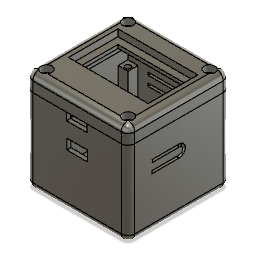
Digital Die v5 (Autodesk Fusion 360 design; units mm, degrees)
Autodesk Fusion 360 part; units mm, degrees
note: some values were not read from the file. Set by a fixed rule: which sketch regions a step uses.
sketch "Sketch1" plane through (0, 0, 0) normal (0, 1, 0) x (1, 0, 0)
  line L0 (0, 0) -> (38.1, 0)
  line L1 (38.1, 0) -> (38.1, 38.1)
  line L2 (38.1, 38.1) -> (0, 38.1)
  line L3 (0, 38.1) -> (0, 0)
  dimension "d1" = 38.1
  dimension "d2" = 38.1
extrude "Extrude1" add sketch "Sketch1" along normal blind 6.35 makes body 1
sketch "Sketch2" plane through (0, 6.35, 0) normal (0, 1, 0) x (-1, 0, 0)
  line L0 (0, -38.1) -> (0, 0)
  line L1 (0, 0) -> (-38.1, 0)
  line L2 (-38.1, 0) -> (-38.1, -38.1)
  line L3 (-38.1, -38.1) -> (0, -38.1)
  line L4 (-6.6675, -27.686) -> (-31.4325, -27.686)
  line L5 (-31.4325, -27.686) -> (-31.4325, -14.224)
  line L6 (-31.4325, -14.224) -> (-6.6675, -14.224)
  line L7 (-6.6675, -14.224) -> (-6.6675, -27.686)
  dimension "d5" = 24.765
  dimension "d6" = 13.462
  measures "d5" distance of L0.end
extrude "Extrude2" cut sketch "Sketch2" against normal blind 6.35 contours L4 L5 L6 L7 bodies 1
sketch "Sketch3" plane through (0, 0, 0) normal (0, -1, 0) x (1, 0, 0)
  line L0 (31.4325, -14.224) -> (31.4325, -27.686)
  line L1 (31.4325, -27.686) -> (6.6675, -27.686)
  line L2 (6.6675, -27.686) -> (6.6675, -14.224)
  line L3 (6.6675, -14.224) -> (31.4325, -14.224)
  line L4 (0, 0) -> (0, -38.1)
  line L5 (0, -38.1) -> (38.1, -38.1)
  line L6 (38.1, -38.1) -> (38.1, 0)
  line L7 (38.1, 0) -> (0, 0)
  line L8 (5.4032, -4.9571) -> (32.8352, -4.9571)
  line L9 (32.8352, -4.9571) -> (32.8352, -32.3891)
  line L10 (32.8352, -32.3891) -> (5.4032, -32.3891)
  line L11 (5.4032, -32.3891) -> (5.4032, -4.9571)
  dimension "d9" = 27.432
  dimension "d10" = 27.432
extrude "Extrude3" cut sketch "Sketch3" against normal blind 2.54 contours L8 L9 L10 L11 bodies 1
sketch "Sketch4" plane through (0, 6.35, 0) normal (0, 1, 0) x (-1, 0, 0)
  line L0 (-31.4325, -27.686) -> (-31.4325, -14.224)
  line L1 (-31.4325, -14.224) -> (-6.6675, -14.224)
  line L2 (-6.6675, -14.224) -> (-6.6675, -27.686)
  line L3 (-6.6675, -27.686) -> (-31.4325, -27.686)
  line L4 (0, -38.1) -> (0, 0)
  line L5 (0, 0) -> (-38.1, 0)
  line L6 (-38.1, 0) -> (-38.1, -38.1)
  line L7 (-38.1, -38.1) -> (0, -38.1)
  line L8 (-4.131, -30.2383) -> (-33.976, -30.2383)
  line L9 (-33.976, -30.2383) -> (-33.976, -11.6963)
  line L10 (-33.976, -11.6963) -> (-4.131, -11.6963)
  line L11 (-4.131, -11.6963) -> (-4.131, -30.2383)
  dimension "d13" = 29.845
  dimension "d14" = 18.542
  measures "d13" distance of L4.end
extrude "Extrude4" cut sketch "Sketch4" against normal blind 2.54 contours L8 L9 L10 L11 bodies 1
sketch "Sketch5" plane through (0, 6.35, 0) normal (0, 1, 0) x (-1, 0, 0)
  line L0 (-33.976, -30.2383) -> (-33.976, -11.6963)
  line L1 (-33.976, -11.6963) -> (-4.131, -11.6963)
  line L2 (-4.131, -11.6963) -> (-4.131, -30.2383)
  line L3 (-4.131, -30.2383) -> (-33.976, -30.2383)
  line L4 (0, -38.1) -> (0, 0)
  line L5 (0, 0) -> (-38.1, 0)
  line L6 (-38.1, 0) -> (-38.1, -38.1)
  line L7 (-38.1, -38.1) -> (0, -38.1)
  circle A0 centre (-3.818, -34.3002) radius 1.016
  circle A1 centre (-3.818, -3.8202) radius 1.016
  circle A2 centre (-34.298, -34.3002) radius 1.016
  circle A3 centre (-34.298, -3.8202) radius 1.016
  dimension "d17" = 2.032
  dimension "d18" = 2.032
  dimension "d19" = 2.032
  dimension "d20" = 2.032
  measures "d17" diameter of A0
  measures "d18" diameter of A1
  measures "d19" diameter of A2
  measures "d20" diameter of A3
fillet "Fillet1" radius 2.54 1 edges at (19.05, 6.35, 0) on bodies 1
fillet "Fillet2" radius 2.54 3 edges at (0, 6.35, -20.32) (0, 5.6061, -0.7439) (0, 1.905, 0) on bodies 1
fillet "Fillet3" radius 2.54 3 edges at (20.32, 6.35, -38.1) (0.7439, 5.6061, -38.1) (0, 1.905, -38.1) on bodies 1
fillet "Fillet4" radius 2.54 5 edges at (38.1, 1.905, 0) (38.1, 5.6061, -0.7439) (38.1, 6.35, -19.05) (38.1, 5.6061, -37.3561) (38.1, 1.905, -38.1) on bodies 1
extrude "Extrude5" cut sketch "Sketch5" against normal blind 6.35 contours A0 | A1 | A2 | A3 bodies 1
sketch "Sketch6" plane through (0, 6.35, 0) normal (0, 1, 0) x (-1, 0, 0)
  circle A0 centre (-34.298, -34.3002) radius 1.016
  circle A1 centre (-34.298, -3.8202) radius 1.016
  circle A2 centre (-3.818, -34.3002) radius 1.016
  circle A3 centre (-3.818, -3.8202) radius 1.016
  line L0 (-33.976, -30.2383) -> (-33.976, -11.6963)
  line L1 (-33.976, -11.6963) -> (-4.131, -11.6963)
  line L2 (-4.131, -11.6963) -> (-4.131, -30.2383)
  line L3 (-4.131, -30.2383) -> (-33.976, -30.2383)
  line L4 (-35.56, -2.54) -> (-35.56, -35.56)
  line L5 (-35.56, -35.56) -> (-2.54, -35.56)
  line L6 (-2.54, -35.56) -> (-2.54, -2.54)
  line L7 (-2.54, -2.54) -> (-35.56, -2.54)
  circle A4 centre (-3.818, -34.3002) radius 2.032
  circle A5 centre (-34.298, -34.3002) radius 2.032
  circle A6 centre (-3.818, -3.8202) radius 2.032
  circle A7 centre (-34.298, -3.8202) radius 2.032
  dimension "d27" = 4.064
  dimension "d28" = 4.064
  dimension "d29" = 4.064
  dimension "d30" = 4.064
  measures "d27" diameter of A4
  measures "d28" diameter of A5
  measures "d29" diameter of A6
  measures "d30" diameter of A7
extrude "Extrude6" cut sketch "Sketch6" against normal blind 2.54 contours L4 L7 A7 | L4 L7 A7 | L4 L5 A5 | L4 L5 A5 | L6 L7 A6 | L6 L7 A6 | L5 L6 A4 | L5 L6 A4 bodies 1
sketch "Sketch1 (2)" plane through (0, 0, 0) normal (0, 1, 0) x (1, 0, 0) in component "Body"
  line L0 (0, 0) -> (38.1, 0)
  line L1 (38.1, 0) -> (38.1, 38.1)
  line L2 (38.1, 38.1) -> (0, 38.1)
  line L3 (0, 38.1) -> (0, 0)
  dimension "d33" = 38.1
  dimension "d34" = 38.1
extrude "Extrude1'" add sketch "Sketch1 (2)" along normal blind 31.75 separate body makes body 2 in component "Body"
shell "Shell1" thickness 1.524 removed faces 1 at (12.7, 31.75, -25.4) on bodies 2 in component "Body"
fillet "Fillet1'" radius 2.54 1 edges at (0, 15.875, 0) on bodies 2 in component "Body"
fillet "Fillet2'" radius 2.54 1 edges at (38.1, 15.875, 0) on bodies 2 in component "Body"
fillet "Fillet3'" radius 2.54 1 edges at (0, 15.875, -38.1) on bodies 2 in component "Body"
fillet "Fillet4'" radius 2.54 1 edges at (38.1, 15.875, -38.1) on bodies 2 in component "Body"
fillet "Fillet5" radius 2.54 8 edges at (19.05, 0, 0) (37.3561, 0, -0.7439) (38.1, 0, -19.05) (37.3561, 0, -37.3561) (19.05, 0, -38.1) (0.7439, 0, -37.3561) (0, 0, -19.05) (0.7439, 0, -0.7439) on bodies 2 in component "Body"
sketch "Sketch2 (2)" plane through (0, 0, 0) normal (0, 0, 1) x (1, 0, 0) in component "Body"
  line L0 (2.54, 2.54) -> (35.56, 2.54)
  line L1 (35.56, 2.54) -> (35.56, 31.75)
  line L2 (35.56, 31.75) -> (2.54, 31.75)
  line L3 (2.54, 31.75) -> (2.54, 2.54)
  line L4 (15.1404, 31.75) -> (22.7604, 31.75)
  line L5 (22.7604, 31.75) -> (22.7604, 28.956)
  line L6 (22.7604, 28.956) -> (15.1404, 28.956)
  line L7 (15.1404, 28.956) -> (15.1404, 31.75)
  dimension "d43" = 7.62
  dimension "d44" = 2.794
  measures "d43" distance of origin
extrude "Extrude2'" cut sketch "Sketch2 (2)" against normal blind 2.54 contours L2 L4 L5 L6 L7 bodies 2 in component "Body"
sketch "Sketch3 (2)" plane through (0, 0, 0) normal (0, 0, 1) x (1, 0, 0) in component "Body"
  line L0 (15.1404, 28.956) -> (15.1404, 31.75)
  line L1 (15.1404, 31.75) -> (2.54, 31.75)
  line L2 (2.54, 31.75) -> (2.54, 2.54)
  line L3 (2.54, 2.54) -> (35.56, 2.54)
  line L4 (35.56, 2.54) -> (35.56, 31.75)
  line L5 (35.56, 31.75) -> (22.7604, 31.75)
  line L6 (22.7604, 31.75) -> (22.7604, 28.956)
  line L7 (22.7604, 28.956) -> (15.1404, 28.956)
  line L8 (15.24, 23.368) -> (22.86, 23.368)
  line L9 (22.86, 23.368) -> (22.86, 19.558)
  line L10 (22.86, 19.558) -> (15.24, 19.558)
  line L11 (15.24, 19.558) -> (15.24, 23.368)
  dimension "d47" = 7.62
  dimension "d48" = 3.81
  measures "d47" distance of origin
extrude "Extrude3'" cut sketch "Sketch3 (2)" against normal blind 2.54 contours L8 L9 L10 L11 bodies 2 in component "Body"
sketch "Sketch4 (2)" plane through (0, 0, 0) normal (-1, 0, 0) x (0, 0, 1) in component "Body"
  line L0 (-35.56, 2.54) -> (-2.54, 2.54)
  line L1 (-2.54, 2.54) -> (-2.54, 31.75)
  line L2 (-2.54, 31.75) -> (-35.56, 31.75)
  line L3 (-35.56, 31.75) -> (-35.56, 2.54)
  arc A0 (-19.2198, 23.367) -> (-19.0834, 18.797) centre (-19.1516, 21.082) ccw
  line L4 (-19.1516, 21.082) -> (-19.2198, 23.367) construction
  line L5 (-19.1516, 21.082) -> (-19.0834, 18.797) construction
  arc A1 (-19.1895, 22.3514) -> (-19.1137, 19.8126) centre (-19.1516, 21.082) ccw
  line L6 (-19.1516, 21.082) -> (-19.1895, 22.3514) construction
  line L7 (-19.1516, 21.082) -> (-19.1137, 19.8126) construction
  line L8 (-19.2198, 23.367) -> (-9.0598, 23.367)
  line L9 (-9.0598, 23.367) -> (-9.0598, 22.3514)
  line L10 (-9.0598, 22.3514) -> (-19.2198, 22.3514)
  line L11 (-19.2198, 22.3514) -> (-19.2198, 23.367)
  line L12 (-19.1137, 19.8126) -> (-8.9537, 19.8126)
  line L13 (-8.9537, 19.8126) -> (-8.9537, 18.797)
  line L14 (-8.9537, 18.797) -> (-19.1137, 18.797)
  line L15 (-19.1137, 18.797) -> (-19.1137, 19.8126)
  dimension "d51" = 2.286
  dimension "d52" = 180
  dimension "d53" = 1.27
  dimension "d54" = 180
  dimension "d55" = 10.16
  dimension "d56" = 10.16
  measures "d51" radius of A0
  measures "d52" angle of L4 L5
  measures "d53" radius of A1
  measures "d54" angle of L6 L7
extrude "Extrude4'" cut sketch "Sketch4 (2)" against normal blind 38.1 contours A0 A1 L11 L15 | A1 L8 L9 L10 L11 | A0 L12 L13 L14 L15 bodies 2 in component "Body"
move_body "Move1" bodies 1 to x (1, 0, 0) y (0, 1, 0) z (0, 0, 1) at (0, 31.75, 0)
sketch "Sketch7" plane through (0, 0, -38.1) normal (0, 0, -1) x (-1, 0, 0)
  line L0 (-35.56, 2.54) -> (-2.54, 2.54)
  line L1 (-2.54, 2.54) -> (-2.54, 31.75)
  line L2 (-2.54, 31.75) -> (-35.56, 31.75)
  line L3 (-35.56, 31.75) -> (-35.56, 2.54)
  arc A0 (-19.1516, 22.352) -> (-19.1516, 19.812) centre (-19.1516, 21.082) ccw
  line L4 (-19.1516, 21.082) -> (-19.1516, 22.352) construction
  line L5 (-19.1516, 21.082) -> (-19.1516, 19.812) construction
  arc A1 (-19.1516, 23.368) -> (-19.1516, 18.796) centre (-19.1516, 21.082) ccw
  line L6 (-19.1516, 21.082) -> (-19.1516, 23.368) construction
  line L7 (-19.1516, 21.082) -> (-19.1516, 18.796) construction
  line L8 (-19.1516, 23.368) -> (-19.1516, 22.352)
  line L9 (-19.1516, 22.352) -> (-8.9916, 22.352)
  line L10 (-8.9916, 22.352) -> (-8.9916, 23.368)
  line L11 (-8.9916, 23.368) -> (-19.1516, 23.368)
  line L12 (-19.1516, 19.812) -> (-19.1516, 18.796)
  line L13 (-19.1516, 18.796) -> (-8.9916, 18.796)
  line L14 (-8.9916, 18.796) -> (-8.9916, 19.812)
  line L15 (-8.9916, 19.812) -> (-19.1516, 19.812)
  dimension "d59" = 1.27
  dimension "d60" = 180
  dimension "d61" = 2.286
  dimension "d62" = 180
  dimension "d63" = 10.16
  dimension "d64" = 10.16
  measures "d59" radius of A0
  measures "d60" angle of L4 L5
  measures "d61" radius of A1
  measures "d62" angle of L6 L7
extrude "Extrude5'" cut sketch "Sketch7" against normal blind 15.24 contours A0 A1 L8 L12 | L8 L9 L10 L11 | L12 L13 L14 L15 bodies 2 in component "Body"
sketch "Sketch8" plane through (0, 0, 0) normal (0, -1, 0) x (1, 0, 0)
  line L0 (35.56, -2.54) -> (2.54, -2.54)
  line L1 (2.54, -2.54) -> (2.54, -35.56)
  line L2 (2.54, -35.56) -> (35.56, -35.56)
  line L3 (35.56, -35.56) -> (35.56, -2.54)
extrude "Extrude6'" add 1 faces at (13.208, 1.524, -13.208) along direction (0, 1, 0) blind 22.098 on bodies 2 bodies 2 in component "Body"
sketch "Sketch9" plane through (0, 23.622, 0) normal (0, 1, 0) x (-1, 0, 0)
  line L0 (-1.524, -36.576) -> (-1.524, -1.524)
  line L1 (-1.524, -1.524) -> (-36.576, -1.524)
  line L2 (-36.576, -1.524) -> (-36.576, -36.576)
  line L3 (-36.576, -36.576) -> (-1.524, -36.576)
  line L4 (-5.2343, -36.576) -> (-32.8695, -36.576)
  line L5 (-32.8695, -36.576) -> (-32.8695, -32.8676)
  line L6 (-32.8695, -32.8676) -> (-5.2343, -32.8676)
  line L7 (-5.2343, -32.8676) -> (-5.2343, -36.576)
  line L8 (-5.2343, -32.8676) -> (-1.524, -32.8676)
  line L9 (-1.524, -32.8676) -> (-1.524, -5.2324)
  line L10 (-1.524, -5.2324) -> (-5.2343, -5.2324)
  line L11 (-5.2343, -5.2324) -> (-5.2343, -32.8676)
  line L12 (-5.2343, -5.2324) -> (-32.8695, -5.2324)
  line L13 (-32.8695, -5.2324) -> (-32.8695, -1.524)
  line L14 (-32.8695, -1.524) -> (-5.2343, -1.524)
  line L15 (-5.2343, -1.524) -> (-5.2343, -5.2324)
  line L16 (-32.8695, -5.2324) -> (-36.576, -5.2324)
  line L17 (-36.576, -5.2324) -> (-36.576, -32.8676)
  line L18 (-36.576, -32.8676) -> (-32.8695, -32.8676)
  line L19 (-32.8695, -32.8676) -> (-32.8695, -5.2324)
  dimension "d79" = 27.6352
  dimension "d80" = 3.7084
  dimension "d81" = 3.7103
  dimension "d82" = 27.6352
  dimension "d83" = 27.6352
  dimension "d84" = 27.6352
  measures "d79" distance of origin
  measures "d84" distance of origin
extrude "Extrude7" cut sketch "Sketch9" against normal blind 22.098 contours L0 L8 L9 L10 L11 | L3 L4 L5 L6 L7 | L6 L11 L12 L19 | L1 L12 L13 L14 L15 | L2 L16 L17 L18 L19 bodies 2 in component "Body"
sketch "Sketch10" plane through (0, 23.622, 0) normal (0, 1, 0) x (-1, 0, 0)
  line L0 (-32.8695, -36.576) -> (-32.8695, -32.8676)
  line L1 (-32.8695, -32.8676) -> (-36.576, -32.8676)
  line L2 (-36.576, -32.8676) -> (-36.576, -36.576)
  line L3 (-36.576, -36.576) -> (-32.8695, -36.576)
  circle A0 centre (-34.298, -34.3002) radius 1.016
  circle A1 centre (-3.818, -34.3002) radius 1.016
  circle A2 centre (-3.8182, -3.8333) radius 1.0159
  circle A3 centre (-34.298, -3.8202) radius 1.016
  dimension "d87" = 2.032
  measures "d87" diameter of A0
extrude "Extrude8" cut sketch "Sketch10" against normal blind 6.35 contours A0 | A1 | A2 | A3 bodies 2 in component "Body"
sketch "Sketch11" plane through (0, 0, 0) normal (0, 1, 0) x (1, 0, 0)
  line L0 (1.5995, 1.5827, 31.75) -> (36.5245, 1.5827, 31.75)
  line L1 (36.5245, 1.5827, 31.75) -> (36.5245, 36.5077, 31.75)
  line L2 (36.5245, 36.5077, 31.75) -> (1.5995, 36.5077, 31.75)
  line L3 (1.5995, 36.5077, 31.75) -> (1.5995, 1.5827, 31.75)
  line L4 (2.543, 2.5334, 31.75) -> (35.563, 2.5334, 31.75)
  line L5 (35.563, 2.5334, 31.75) -> (35.563, 35.5534, 31.75)
  line L6 (35.563, 35.5534, 31.75) -> (2.543, 35.5534, 31.75)
  line L7 (2.543, 35.5534, 31.75) -> (2.543, 2.5334, 31.75)
sketch "Sketch11 (curves 31.75 mm off its plane)" plane through (0, 31.75, 0) normal (0, 1, 0) x (1, 0, 0)
  line L0 (1.5995, 1.5827) -> (36.5245, 1.5827)
  line L1 (36.5245, 1.5827) -> (36.5245, 36.5077)
  line L2 (36.5245, 36.5077) -> (1.5995, 36.5077)
  line L3 (1.5995, 36.5077) -> (1.5995, 1.5827)
  line L4 (2.543, 2.5334) -> (35.563, 2.5334)
  line L5 (35.563, 2.5334) -> (35.563, 35.5534)
  line L6 (35.563, 35.5534) -> (2.543, 35.5534)
  line L7 (2.543, 35.5534) -> (2.543, 2.5334)
extrude "Extrude7'" add sketch "Sketch11 (curves 31.75 mm off its plane)" against normal blind 2.54 bodies 1
fillet "Fillet5'" radius 1.27 1 edges at (1.5995, 30.48, -1.5827) on bodies 1
fillet "Fillet6" radius 1.27 1 edges at (36.5245, 30.48, -1.5827) on bodies 1
fillet "Fillet7" radius 1.27 1 edges at (36.5245, 30.48, -36.5077) on bodies 1
fillet "Fillet8" radius 1.27 1 edges at (1.5995, 30.48, -36.5077) on bodies 1
sketch "Sketch12" plane through (0, 0, -1.5827) normal (0, 0, 1) x (1, 0, 0)
  line L0 (35.2545, 29.21) -> (35.2545, 31.75)
  line L1 (35.2545, 31.75) -> (2.8695, 31.75)
  line L2 (2.8695, 31.75) -> (2.8695, 29.21)
  line L3 (2.8695, 29.21) -> (35.2545, 29.21)
  line L4 (15.1404, 31.75) -> (22.7604, 31.75)
  line L5 (22.7604, 31.75) -> (22.7604, 28.956)
  line L6 (22.7604, 28.956) -> (15.1404, 28.956)
  line L7 (15.1404, 28.956) -> (15.1404, 31.75)
extrude "Extrude8'" cut sketch "Sketch12" against normal blind 2.54 contours L1 L3 L4 L5 L7 bodies 1
component "Body" placed x (1, 0, 0) y (0, 1, 0) z (0, 0, 1) at (0, 0, 0)
